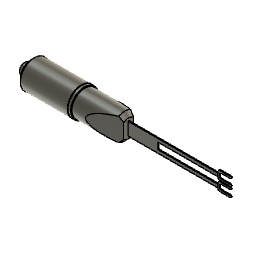
Ballon caneta externo v1 (Autodesk Fusion 360 design; units mm, degrees)
Autodesk Fusion 360 part; units mm, degrees
sketch "Sketch1" plane through (0, 0, 0) normal (0, 1, 0) x (1, 0, 0)
  line L0 (0, 0) -> (10, 0)
  line L1 (10, 0) -> (10, -5)
  line L2 (10, -5) -> (0, -5)
  line L3 (0, -5) -> (0, 0)
  line L4 (10, 0) -> (50, 0)
  line L5 (50, 0) -> (50, -6.5)
  line L6 (50, -6.5) -> (10, -6.5)
  line L7 (10, -6.5) -> (10, 0)
  line L8 (50, 0) -> (65, 0)
  line L9 (65, 0) -> (65, -3.25)
  line L10 (65, -3.25) -> (50, -3.25)
  line L11 (50, -3.25) -> (50, 0)
  line L12 (65, -3.25) -> (95, -3.25)
  line L13 (95, -3.25) -> (95, -1.625)
  line L14 (95, -1.625) -> (65, -1.625)
  line L15 (65, -1.625) -> (65, -3.25)
  line L16 (50, 0) -> (65, 0)
  line L17 (65, 0) -> (65, 3.25)
  line L18 (65, 3.25) -> (50, 3.25)
  line L19 (50, 3.25) -> (50, 0)
  line L20 (65, 1.625) -> (95, 1.625)
  line L21 (95, 1.625) -> (95, 3.25)
  line L22 (95, 3.25) -> (65, 3.25)
  line L23 (65, 3.25) -> (65, 1.625)
  line L24 (96, 0.2457) -> (101.3215, 0.2457)
  line L25 (101.8215, 0.7457) -> (101.8215, 0.6225)
  line L26 (101.3215, 4.6297) -> (96, 4.6297)
  line L27 (95, 3.6297) -> (95, 1.2457)
  line L28 (101.3215, 1.1225) -> (96.8215, 1.1225)
  line L29 (95.8215, 2.1225) -> (95.8215, 2.6962)
  line L30 (96.8215, 3.6962) -> (101.3215, 3.6962)
  arc A0 (95, 1.2457) -> (96, 0.2457) centre (96, 1.2457) ccw
  arc A1 (95.8215, 2.1225) -> (96.8215, 1.1225) centre (96.8215, 2.1225) ccw
  arc A2 (96, 4.6297) -> (95, 3.6297) centre (96, 3.6297) ccw
  arc A3 (96.8215, 3.6962) -> (95.8215, 2.6962) centre (96.8215, 2.6962) ccw
  arc A4 (101.3215, 0.2457) -> (101.8215, 0.7457) centre (101.3215, 0.7457) ccw
  arc A5 (101.8215, 0.6225) -> (101.3215, 1.1225) centre (101.3215, 0.6225) ccw
  line L31 (101.8215, 4.1962) -> (101.8215, 4.1297)
  arc A6 (101.3215, 3.6962) -> (101.8215, 4.1962) centre (101.3215, 4.1962) ccw
  arc A7 (101.8215, 4.1297) -> (101.3215, 4.6297) centre (101.3215, 4.1297) ccw
  arc A8 (101.8215, -0.7457) -> (101.3215, -0.2457) centre (101.3215, -0.7457) ccw
  arc A9 (101.3215, -1.1225) -> (101.8215, -0.6225) centre (101.3215, -0.6225) ccw
  line L32 (101.3215, -1.1225) -> (96.8215, -1.1225)
  line L33 (96, -0.2457) -> (101.3215, -0.2457)
  arc A10 (96, -0.2457) -> (95, -1.2457) centre (96, -1.2457) ccw
  arc A11 (96.8215, -1.1225) -> (95.8215, -2.1225) centre (96.8215, -2.1225) ccw
  line L34 (95, -3.6297) -> (95, -1.2457)
  arc A12 (95, -3.6297) -> (96, -4.6297) centre (96, -3.6297) ccw
  arc A13 (95.8215, -2.6962) -> (96.8215, -3.6962) centre (96.8215, -2.6962) ccw
  line L35 (95.8215, -2.1225) -> (95.8215, -2.6962)
  line L36 (96.8215, -3.6962) -> (101.3215, -3.6962)
  line L37 (101.3215, -4.6297) -> (96, -4.6297)
  arc A14 (101.3215, -4.6297) -> (101.8215, -4.1297) centre (101.3215, -4.1297) ccw
  arc A15 (101.8215, -4.1962) -> (101.3215, -3.6962) centre (101.3215, -4.1962) ccw
  point P0 (101.8215, 1.1225)
  point P1 (95.8215, 1.1225)
  dimension "d1" = 10
  dimension "d2" = 5
  dimension "d3" = 40
  dimension "d4" = 6.5
  dimension "d5" = 15
  dimension "d6" = 30
  dimension "d7" = 3.25
  dimension "d8" = 30
  dimension "d9" = 6
  dimension "d10" = 1
  dimension "d11" = 0.5
  dimension "d12" = 0.5
  constraint horizontal L0
  constraint vertical L1
  constraint horizontal L2
  constraint vertical L3
  constraint coincident L0.start L3.end
  constraint horizontal L4
  constraint vertical L5
  constraint horizontal L6
  constraint vertical L7
  constraint horizontal L8
  constraint vertical L9
  constraint horizontal L10
  constraint vertical L11
  constraint horizontal L12
  constraint vertical L13
  constraint horizontal L14
  constraint vertical L15
  constraint horizontal L16
  constraint vertical L17
  constraint horizontal L18
  constraint vertical L19
  constraint horizontal L20
  constraint vertical L21
  constraint horizontal L22
  constraint vertical L23
  constraint midpoint L17 L20.start
  constraint horizontal L24
  constraint vertical L25
  constraint horizontal L26
  constraint vertical L27
  constraint coincident L25 P0
  constraint perpendicular L25 L28
  constraint perpendicular L26 L29
  constraint perpendicular L25 L30
  constraint tangent L24 A0
  constraint tangent L27 A0
  constraint coincident P1 L28
  constraint coincident P1 L29
  constraint tangent L28 A1
  constraint tangent L29 A1
  constraint equal A0 A1
  constraint tangent L26 A2
  constraint tangent L27 A2
  constraint equal A0 A2
  constraint tangent L29 A3
  constraint tangent L30 A3
  constraint equal A0 A3
  constraint tangent L24 A4
  constraint tangent L25 A4
  constraint coincident P0 L28
  constraint tangent L28 A5
  constraint tangent L25 A5
  constraint equal A4 A5
  constraint perpendicular L26 L31
  constraint tangent L30 A6
  constraint tangent L31 A6
  constraint tangent L26 A7
  constraint tangent L31 A7
  constraint equal A6 A7
  measures "d1" distance of L0.start L0.end
  measures "d2" distance of L0.start L2.end
  measures "d3" distance of L0.end L4.end
  measures "d4" distance of L0.end L6.end
  measures "d5" distance of L4.end L8.end
  measures "d6" distance of L9.end L12.end
  measures "d7" distance of L4.end L18.end
  measures "d8" distance of L20.start L20.end
  measures "d9" distance of P0 P1
  measures "d10" radius of A0
  measures "d11" radius of A4
  measures "d12" radius of A6
revolve "Revolve1" add sketch "Sketch1" angle 360 about axis through (10, 0, 0) along (1, 0, 0) contours L0 L1 L2 L3 L7 | L1 L4 L5 L6 L7 L11 makes body 1
extrude "Extrude1" add sketch "Sketch1" along normal mid plane 0.5 contours L5 L8 L9 L10 L11 L15 L16 | L8 L16 L17 L18 L19 L23 | L9 L12 L13 L14 L15 L34 | L17 L20 L21 L22 L23 L27 bodies 1
extrude "Extrude2" add sketch "Sketch1" along normal blind 0.5 contours L13 A8 A9 L32 L33 A10 A11 L34 A12 A13 L35 L36 L37 A14 A15 | L21 L24 L26 L27 L28 L29 L30 A0 A1 A2 A3 A4 A5 A6 A7 bodies 1
thread "Thread1" "AFBMA Standard Locknuts 0.391 N 00 3A" major diameter 9.8628 minor diameter 8.9586 pitch 0.7937 angle 60 modelled right hand crest width 0.1197 on face at (6.6667, 0.2492, 4.9938) crest through (10.1984, 0, 4.9314) on bodies 1
hole "Hole1" at (0, 0, 0) direction (1, 0, 0) diameter 8 depth 36 tip angle 180 bodies 1
sketch "Sketch2" plane through (0, 0, 0) normal (0, 0, 1) x (1, 0, 0)
  line L0 (27.8607, 8.7744) -> (-2.4928, 8.7744)
  line L1 (-2.4928, 8.7744) -> (-2.4928, -10.9554)
  line L2 (-2.4928, -10.9554) -> (27.8607, -10.9554)
  line L3 (27.8607, -10.9554) -> (27.8607, 8.7744)
  constraint horizontal L0
  constraint vertical L1
  constraint horizontal L2
  constraint vertical L3
extrude "Extrude3" cut sketch "Sketch2" along normal mid plane 40 bodies 1
sketch "Sketch3" plane through (27.8607, 0, 0) normal (-1, 0, 0) x (0, -1, 0)
  circle A0 centre (0, 0) radius 4
  circle A1 centre (0, 0) radius 6.5
  circle A2 centre (0, 0) radius 7
  dimension "d23" = 14
  constraint coincident A0.centre A1.centre
  measures "d23" diameter of A2
extrude "Extrude4" add sketch "Sketch3" along normal blind 1.5 contours A0 | A1 | A2 bodies 1
sketch "Sketch4" plane through (0, 0, 0) normal (0, 0, 1) x (1, 0, 0)
  line L0 (26.1566, 7.0871) -> (2.4888, 7.0871)
  line L1 (2.4888, 7.0871) -> (2.4888, 0)
  line L2 (2.4888, 0) -> (26.1566, 0)
  line L3 (26.1566, 0) -> (26.1566, 7.0871)
  line L4 (2.4888, 0) -> (0.9815, 0)
  line L5 (0.9815, 0) -> (0.9815, 5.6814)
  line L6 (0.9815, 5.6814) -> (2.4888, 5.6814)
  line L7 (2.4888, 5.6814) -> (2.4888, 0)
  line L8 (0.9815, 0) -> (-0.1148, 0)
  line L9 (-0.1148, 0) -> (-0.1148, 3.5435)
  line L10 (-0.1148, 3.5435) -> (0.9815, 3.5435)
  line L11 (0.9815, 3.5435) -> (0.9815, 0)
  line L12 (0, 0) -> (-2.4444, 0)
  line L13 (-2.4444, 0) -> (-2.4444, 2.6667)
  line L14 (-2.4444, 2.6667) -> (0, 2.6667)
  line L15 (0, 2.6667) -> (0, 0)
  constraint horizontal L0
  constraint vertical L1
  constraint horizontal L2
  constraint vertical L3
  constraint horizontal L4
  constraint vertical L5
  constraint horizontal L6
  constraint vertical L7
  constraint horizontal L8
  constraint vertical L9
  constraint horizontal L10
  constraint vertical L11
  constraint horizontal L12
  constraint vertical L13
  constraint horizontal L14
  constraint vertical L15
  constraint coincident L12.start L15.end
revolve "Revolve2" add sketch "Sketch4" angle 360 about axis through (2.4888, 0, 0) along (1, 0, 0) separate body contours L0 L1 L2 L3 L7 | L1 L4 L5 L6 L7 L11 | L5 L8 L9 L10 L11 L14 L15 | L9 L12 L13 L14 makes body 2
fillet "Fillet1" radius 0.1 3 edges at (0.9815, -2.0545, 5.297) (-0.1148, -1.2814, 3.3037) (-2.4444, -0.9643, 2.4863) on bodies 2
fillet "Fillet2" radius 0.1 1 edges at (27.8607, 6.5263, -2.5313) on bodies 1
chamfer "Chamfer1" distance 2 angle 45 1 edges at (50, -2.3505, -6.0601) on bodies 1
sketch "Sketch5" plane through (0, 0, 0) normal (0, 0, 1) x (1, 0, 0)
  line L0 (49.9491, -6.8357) -> (33.5659, -6.8357)
  line L1 (33.5659, -6.8357) -> (50.7066, -2.2429)
  line L2 (33.5659, -6.8357) -> (50.3973, -6.8357) construction
  line L3 (50.3973, -6.8357) -> (49.9491, -6.8357)
  line L4 (50.3973, -6.8357) -> (50.7066, -2.2429)
  line L5 (50.1732, 0.0034) -> (35.7962, 0.0034)
  line L6 (33.5659, 6.8425) -> (50.3973, 6.8425) construction
  line L7 (49.9491, 6.8425) -> (33.5659, 6.8425)
  line L8 (50.3973, 6.8425) -> (49.9491, 6.8425)
  line L9 (50.3973, 6.8425) -> (50.7066, 2.2496)
  line L10 (33.5659, 6.8425) -> (50.7066, 2.2496)
  dimension "d32" = 15
  constraint horizontal L0
  constraint horizontal L2
  constraint parallel L3 L5
  constraint symmetric L0.start L5 L7.start
  constraint symmetric L0.end L5 L6.start
  constraint symmetric L1.end L5 L9.end
  constraint symmetric L2.end L5 L6.end
  measures "d32" angle of L1 L2
extrude "Extrude6" cut sketch "Sketch5" along normal mid plane 40 bodies 1
extrude "Extrude5" cut sketch "Sketch5" along normal mid plane 40 contours L0 L1 L3 L4 bodies 1
